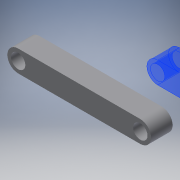
# Autodesk Inventor part: L1
Saved by Autodesk Inventor 2019 (Build 230136000, 136)
## iProperties
Created: 2020-03-18
Part Number: L1
Material: Generic
Document SubType Name: Modeling
Designer: Pulag
Density: 1 g/cm^3
Appearance: Default
Author: Pulag
Autodesk Inventor part; units mm, degrees
ref_plane "YZ Plane" through (0, 0, 0) normal (1, 0, 0) x (0, 1, 0)
ref_plane "XZ Plane" through (0, 0, 0) normal (0, 1, 0) x (-1, 0, 0)
ref_plane "XY Plane" through (0, 0, 0) normal (0, 0, 1) x (1, 0, 0)
sketch "Sketch1" plane through (0, 0, 0) normal (0, 0, 1) x (1, 0, 0)
  line L0 (0, 0) -> (150, 0)
  line L1 (150, 3) -> (0, 3)
  arc A0 (0, 3) -> (0, 0) centre (0, 1.5) ccw
  arc A1 (150, 0) -> (150, 3) centre (150, 1.5) ccw
  circle A2 centre (0, 1.5) radius 1
  circle A3 centre (150, 1.5) radius 1
  line L2 (0, 3) -> (0, 0)
  line L3 (150, 3) -> (150, 0)
  dimension "d2" = 2
  dimension "d3" = 2
  dimension "d9" = 150
  constraints: 8 end point, 4 centre point, 4 point on circle, 2 coincident, 2 parallel, 1 horizontal, 1 vertical
  measures "d2" diameter of A2
  measures "d3" diameter of A3
  measures "d9" distance between parallel lines of L3 L2
extrude "Extrusion1" add sketch "Sketch1" along normal blind 3 contours L2 A2 L1 L3 A3 L0 | A0 L2 A2 | L3 A3 A1
body "Solid1"
